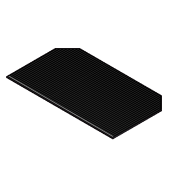
# Autodesk Inventor part: SpaceQuest_UTJ_2
Saved by Autodesk Inventor 2014 (Build 180170000, 170)
## iProperties
Created: 2013-06-08
Part Number: SpaceQuest_UTJ_2
Document SubType Name: Modeling
Designer: Robert Davis
Density: 1 g/cm^3
Material: Generic
Appearance: Default
Author: Robert Davis
Autodesk Inventor part; units mm, degrees
ref_plane "YZ Plane" through (0, 0, 0) normal (1, 0, 0) x (0, 1, 0)
ref_plane "XZ Plane" through (0, 0, 0) normal (0, 1, 0) x (-1, 0, 0)
ref_plane "XY Plane" through (0, 0, 0) normal (0, 0, 1) x (1, 0, 0)
sketch "Sketch1" plane through (0, 0, 0) normal (0, 0, 1) x (1, 0, 0)
  line L0 (-34.555, -19.85) -> (34.555, -19.85)
  line L1 (34.555, -19.85) -> (34.555, 19.85)
  line L2 (34.555, 19.85) -> (-34.555, 19.85)
  line L3 (-34.555, 19.85) -> (-34.555, -19.85)
  line L4 (0, 0) -> (18.4277, 0)
  line L5 (0, 0) -> (0, 21.1115)
  dimension "d0" = 69.11
  dimension "d1" = 39.7
  constraints: 12 end point, 3 horizontal, 3 vertical, 1 coincident, 2 other
  measures "d0" distance of L1.end L2.end
  measures "d1" distance of L0.end L1.end
extrude "Extrusion1" add sketch "Sketch1" along normal blind 0.76
chamfer "Chamfer1" distance 7.87 angle 45 2 edges at (34.555, 19.85, 0.38) (-34.555, 19.85, 0.38)
sketch "Sketch2" plane through (0, 0, 0.76) normal (0, 0, 1) x (1, 0, 0)
  line L0 (-34.555, -19.85) -> (-34.555, 11.98) projected
  line L1 (34.555, -19.85) -> (-34.555, -19.85) projected
  line L2 (34.555, 11.98) -> (34.555, -19.85) projected
  line L3 (-26.685, 19.85) -> (26.685, 19.85) projected
  line L4 (-34.4594, 20.0154) -> (34.555, 19.85) construction
  line L5 (34.555, 19.85) -> (34.4594, -20.0154) construction
  line L6 (34.4594, -20.0154) -> (-34.555, -19.85) construction
  line L7 (-34.555, -19.85) -> (-34.4594, 20.0154) construction
  point P0 (0, 0)
  constraints: 4 point on line, 2 other
decal "Decal1"
body "Solid1"
